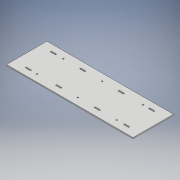
# Autodesk Inventor part: PISO
Saved by Autodesk Inventor 2018 (Build 220112000, 112)
## iProperties
Created: 2018-03-05
Part Number: PISO
Material: Generic
Document SubType Name: Modeling
Designer: isai
Density: 1 g/cm^3
Appearance: Default
Author: isai
Autodesk Inventor part; units mm, degrees
ref_plane "YZ Plane" through (0, 0, 0) normal (1, 0, 0) x (0, 1, 0)
ref_plane "XZ Plane" through (0, 0, 0) normal (0, 1, 0) x (-1, 0, 0)
ref_plane "XY Plane" through (0, 0, 0) normal (0, 0, 1) x (1, 0, 0)
sketch "Sketch1" plane through (0, 0, 0) normal (0, 0, 1) x (1, 0, 0)
  line L0 (20, 0) -> (0, 0)
  line L1 (20, -4) -> (0, -4)
  line L2 (20, 0) -> (20, -4)
  line L3 (0, 0) -> (0, -4)
  line L4 (45, -4) -> (45, 0)
  line L5 (48.6, 0) -> (48.6, -4)
  line L6 (4.5603, -97.794) -> (24.5603, -97.794)
  line L7 (4.5603, -101.794) -> (24.5603, -101.794)
  line L8 (24.5603, -101.794) -> (24.5603, -97.794)
  line L9 (4.5603, -101.794) -> (4.5603, -97.794)
  line L10 (45, -101.794) -> (45, -97.794)
  line L11 (48.6, -97.794) -> (48.6, -101.794)
  line L12 (117.8484, -101.794) -> (117.8484, -97.794)
  line L13 (137.8484, -101.794) -> (137.8484, -97.794)
  line L14 (117.8484, -97.794) -> (137.8484, -97.794)
  line L15 (137.8484, -101.794) -> (117.8484, -101.794)
  line L16 (129.1, 0) -> (109.1, 0)
  line L17 (129.1, -4) -> (109.1, -4)
  line L18 (189.6, -4) -> (189.6, 0)
  line L19 (193.2, 0) -> (193.2, -4)
  line L20 (196.8, -101.794) -> (196.8, -97.794)
  line L21 (200.4, -97.794) -> (200.4, -101.794)
  line L22 (252.1516, 0) -> (252.1516, -4)
  line L23 (272.1516, 0) -> (272.1516, -4)
  line L24 (260.9, -101.794) -> (260.9, -97.794)
  line L25 (280.9, -101.794) -> (280.9, -97.794)
  line L26 (341.4, -4) -> (341.4, 0)
  line L27 (345, 0) -> (345, -4)
  line L28 (341.4, -101.794) -> (341.4, -97.794)
  line L29 (345, -97.794) -> (345, -101.794)
  line L30 (365.4397, 0) -> (365.4397, -4)
  line L31 (385.4397, 0) -> (385.4397, -4)
  line L32 (370, -101.794) -> (370, -97.794)
  line L33 (390, -101.794) -> (390, -97.794)
  line L34 (45, 0) -> (48.6, 0)
  line L35 (45, -4) -> (48.6, -4)
  line L36 (109.1, 0) -> (109.1, -4)
  line L37 (129.1, 0) -> (129.1, -4)
  line L38 (189.6, 0) -> (193.2, 0)
  line L39 (189.6, -4) -> (193.2, -4)
  line L40 (252.1516, 0) -> (272.1516, 0)
  line L41 (252.1516, -4) -> (272.1516, -4)
  line L42 (341.4, 0) -> (345, 0)
  line L43 (341.4, -4) -> (345, -4)
  line L44 (365.4397, 0) -> (385.4397, 0)
  line L45 (365.4397, -4) -> (385.4397, -4)
  line L46 (45, -97.794) -> (48.6, -97.794)
  line L47 (45, -101.794) -> (48.6, -101.794)
  line L48 (196.8, -97.794) -> (200.4, -97.794)
  line L49 (196.8, -101.794) -> (200.4, -101.794)
  line L50 (260.9, -97.794) -> (280.9, -97.794)
  line L51 (260.9, -101.794) -> (280.9, -101.794)
  line L52 (370, -97.794) -> (390, -97.794)
  line L53 (370, -101.794) -> (390, -101.794)
  line L54 (4.5603, -101.794) -> (0, -101.794)
  line L55 (-40, 24.103) -> (430, 24.103)
  line L56 (430, 24.103) -> (430, -125.897)
  line L57 (430, -125.897) -> (-40, -125.897)
  line L58 (-40, -125.897) -> (-40, 24.103)
  line L59 (-40, 24.103) -> (430, -125.897) construction
  line L60 (430, 24.103) -> (-40, -125.897) construction
  line L61 (430, 24.103) -> (280, 24.103)
  line L62 (280, 24.103) -> (280, 124.103)
  line L63 (280, 124.103) -> (430, 124.103)
  line L64 (430, 124.103) -> (430, 24.103)
  line L65 (341.4, -97.794) -> (345, -97.794)
  line L66 (390, -101.794) -> (370, -101.794)
  line L67 (345, -101.794) -> (341.4, -101.794)
  point P0 (195, -50.897)
  dimension "d0" = 470
  dimension "d1" = 150
  dimension "d2" = 150
  dimension "d3" = 100
  constraints: 136 end point, 16 parallel, 10 horizontal, 4 perpendicular, 2 midpoint, 2 vertical, 1 point on line
  measures "d0" distance of L57.start L57.end
  measures "d1" distance of L55.end L57.start
  measures "d2" distance of L62.end L64.start
  measures "d3" distance of L61.end L62.end
extrude "Extrusion1" add sketch "Sketch1" along normal blind 4 contours L55 L56 L57 L58
body "Solid1"
